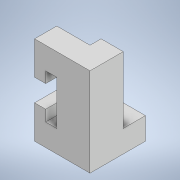
# Autodesk Inventor part: Martin-Probst-26673_obrazek_2
Saved by Autodesk Inventor 2021 (Build 250183000, 183)
## iProperties
Created: 2022-03-18
Part Number: Martin-Probst-26673_obrazek_2
Material: Všeobecné
Document SubType Name: Modeling
Designer: 26673
Density: 1 g/cm^3
Appearance: Výchozí
Author: 26673
Autodesk Inventor part; units mm, degrees
ref_plane "YZ Plane" through (0, 0, 0) normal (1, 0, 0) x (0, 1, 0)
ref_plane "XZ Plane" through (0, 0, 0) normal (0, 1, 0) x (-1, 0, 0)
ref_plane "XY Plane" through (0, 0, 0) normal (0, 0, 1) x (1, 0, 0)
sketch "Náčrt1" plane through (0, 0, 0) normal (1, 0, 0) x (0, 1, 0)
  line L0 (0, 0) -> (0, -50)
  line L1 (0, -50) -> (80, -50)
  line L2 (80, -50) -> (80, 0)
  line L3 (80, 0) -> (0, 0)
  dimension "d0" = 50
  dimension "d1" = 80
  constraints: 8 end point, 3 perpendicular, 1 vertical
  measures "d0" distance of L0.start L0.end
  measures "d1" distance of L0.end L1.end
extrude "Vysunutí1" add sketch "Náčrt1" along normal blind 50
sketch "Náčrt2" plane through (0, 0, -50) normal (0, 0, -1) x (-1, 0, 0)
  line L0 (-50, 0) -> (-50, 80) projected
  line L1 (-50, 0) -> (-50, 20)
  line L2 (-50, 20) -> (-30, 20)
  line L3 (-30, 20) -> (-30, 0)
  line L4 (0, 0) -> (-50, 0) projected
  line L5 (-30, 0) -> (-50, 0)
  line L6 (-50, 0) -> (-50, 80)
  line L7 (-50, 80) -> (-30, 80)
  line L8 (0, 80) -> (-50, 80) projected
  line L9 (-30, 80) -> (-30, 20)
  dimension "d4" = 20
  dimension "d5" = 20
  dimension "d6" = 20
  constraints: 14 end point, 4 perpendicular, 3 point on line
  measures "d4" distance of L0.start L1.end
  measures "d5" distance of L1.end L2.end
  measures "d6" distance of L6.end L7.end
extrude "Vysunutí2" cut sketch "Náčrt2" against normal blind 20 contours L0 L7 L9 L2
sketch "Náčrt3" plane through (0, 0, -50) normal (0, 0, -1) x (-1, 0, 0)
  line L0 (0, 80) -> (-50, 80) projected
  line L1 (0, 0) -> (0, 80) projected
  line L2 (0, 80) -> (0, 0)
  line L3 (0, 0) -> (-30, 0)
  line L4 (0, 0) -> (-50, 0) projected
  line L5 (-30, 0) -> (-30, 80)
  dimension "d9" = 30
  constraints: 6 end point, 1 perpendicular, 1 point on line, 1 vertical
  measures "d9" distance of L1.start L3.end
extrude "Vysunutí3" cut sketch "Náčrt3" against normal blind 30
sketch "Náčrt4" plane through (0, 0, -20) normal (0, 0, -1) x (-1, 0, 0)
  line L0 (0, 80) -> (0, 0) projected
  line L1 (0, 40) -> (0, 30)
  line L2 (0, 30) -> (0, 50)
  line L3 (0, 50) -> (-10, 50)
  line L4 (0, 40) -> (-20, 40)
  line L5 (-20, 40) -> (-20, 60)
  line L6 (-20, 60) -> (-10, 60)
  line L7 (-10, 50) -> (-10, 60)
  line L8 (0, 30) -> (-10, 30)
  dimension "d12" = 10
  dimension "d13" = 20
  dimension "d14" = 10
  dimension "d15" = 20
  dimension "d16" = 20
  dimension "d17" = 10
  constraints: 16 end point, 4 perpendicular, 2 point on line, 1 horizontal, 1 midpoint, 1 vertical
  measures "d12" distance of L1.start L1.end
  measures "d13" distance of L1.end L2.end
  measures "d14" distance of L2.end L3.end
  measures "d15" distance of L1.start L4.end
  measures "d16" distance of L4.end L5.end
  measures "d17" distance of L1.end L8.end
extrude "Vysunutí4" cut sketch "Náčrt4" against normal blind 30
sketch "Náčrt5" plane through (0, 0, -20) normal (0, 0, -1) x (-1, 0, 0)
  line L0 (0, 40) -> (0, 0) projected
  line L1 (-20, 40) -> (-20, 60) projected
  line L2 (0, 40) -> (-20, 40)
  line L3 (-20, 40) -> (-20, 20)
  line L4 (-20, 20) -> (-10, 20)
  line L5 (-10, 20) -> (-10, 30)
  line L6 (-10, 30) -> (0, 30)
  line L7 (0, 40) -> (0, 0) projected
  line L8 (0, 30) -> (0, 40)
  dimension "d20" = 20
  dimension "d21" = 10
  dimension "d22" = 10
  constraints: 12 end point, 5 perpendicular, 1 horizontal
  measures "d20" distance of L1.start L3.end
  measures "d21" distance of L3.end L4.end
  measures "d22" distance of L4.end L5.end
extrude "Vysunutí5" cut sketch "Náčrt5" against normal blind 30
